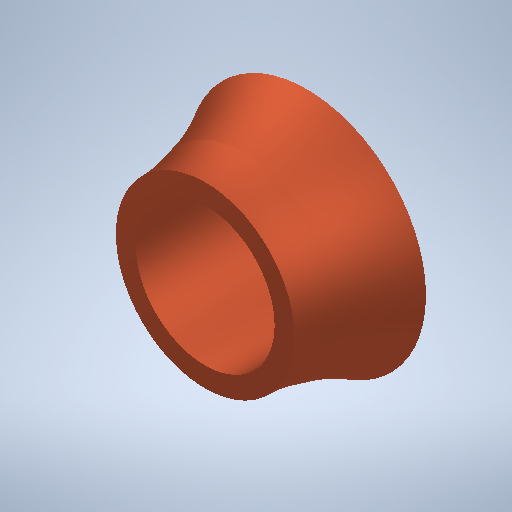
# Autodesk Inventor part: VenturiEinsatz
Saved by Autodesk Inventor 2025 (Build 290162010, 162A)
## iProperties
Created: 2024-07-17
Part Number: VenturiEinsatz
Material: Copper
Document SubType Name: Modeling
Designer: ffogue
Density: 8.94 g/cm^3
Appearance: Copper - Satin
Author: ffogue
Autodesk Inventor part; units mm, degrees
note: some values were not read from the file. Chosen so that the rebuilt part matches the saved one: direction of "Hole1".
ref_plane "YZ Plane" through (0, 0, 0) normal (1, 0, 0) x (0, 1, 0)
ref_plane "XZ Plane" through (0, 0, 0) normal (0, 1, 0) x (-1, 0, 0)
ref_plane "XY Plane" through (0, 0, 0) normal (0, 0, 1) x (1, 0, 0)
sketch "Sketch1" plane through (0, 0, 0) normal (0, 1, 0) x (-1, 0, 0)
  line L0 (0, 0) -> (0, -8)
  line L1 (0, 0) -> (-4.5, 0)
  arc A0 (-4.7918, -2) -> (-4.5, 0) centre (-11.5, 0) ccw
  line L2 (-6, -5.1202) -> (0, -5.1202)
  arc A1 (-6, -5.1202) -> (-4.7918, -2) centre (-14.5898, 0) ccw
  dimension "d6" = 8
  dimension "d7" = 7
  dimension "d9" = 12
  dimension "d10" = 9
  dimension "d11" = 10
  dimension "d12" = 2
  constraints: 6 end point, 4 point on circle, 2 centre point, 2 horizontal alignment, 1 horizontal, 1 perpendicular, 1 point on line, 1 vertical
  measures "d6" distance of L0.start L0.end
  measures "d7" radius of A0
  measures "d9" diameter of L2.start L0
  measures "d10" diameter of L1.end L0
  measures "d11" radius of A1
  measures "d12" vertical distance of A0.start L1.end
revolve "Revolution1" add sketch "Sketch1" angle 360 about axis through (0, 0, 0) along (0, 0, -1)
sketch "Sketch2" plane through (0, 0, 0) normal (0, 0, 1) x (1, 0, 0)
  circle A0 centre (0, 0) radius 4.5 construction
  constraints: 1 coincident
hole "Hole1" at (0, 0, 0) direction (0, 0, -1) diameter 7 depth 5.1202
fillet "Fillet1" radius 1 1 edges at (-4.7918, 0, -2)
body "Solid1"
